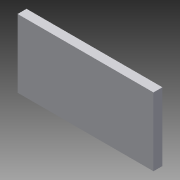
# Autodesk Inventor part: Lapangan2
Saved by Autodesk Inventor 2015 (Build 190159000, 159)
## iProperties
Created: 2015-01-29
Part Number: Lapangan2
Material: Generic
Document SubType Name: Modeling
Designer: Rafi Kurnia Putra
Density: 1 g/cm^3
Appearance: White
Author: Rafi Kurnia Putra
Autodesk Inventor part; units mm, degrees
ref_plane "YZ Plane" through (0, 0, 0) normal (1, 0, 0) x (0, 1, 0)
ref_plane "XZ Plane" through (0, 0, 0) normal (0, 1, 0) x (-1, 0, 0)
ref_plane "XY Plane" through (0, 0, 0) normal (0, 0, 1) x (1, 0, 0)
sketch "Sketch1" plane through (0, 0, 0) normal (0, 1, 0) x (-1, 0, 0)
  line L0 (2430, 1220) -> (0, 1220)
  line L1 (0, -1220) -> (2430, -1220)
  line L2 (2430, -1220) -> (2430, 1220)
  line L3 (2410, 1200) -> (2410, -1200)
  line L4 (10, 650) -> (10, 1200)
  line L5 (740, 150) -> (0, 150)
  line L6 (730, 170) -> (730, 740)
  line L7 (730, 740) -> (750, 740)
  line L8 (750, 740) -> (750, 150)
  line L9 (750, 150) -> (740, 150)
  line L10 (1210, 740) -> (1210, 270)
  line L11 (1230, 290) -> (1230, 740)
  line L12 (1230, 740) -> (1210, 740)
  line L13 (270, 630) -> (270, 650)
  line L14 (10, 1200) -> (2410, 1200)
  line L15 (0, -330) -> (10, -330)
  line L16 (0, -330) -> (10, -330) construction
  line L17 (10, -330) -> (10, -1200)
  line L18 (730, -1200) -> (730, -330)
  line L19 (750, -1200) -> (1600, -1200) construction
  line L20 (730, -330) -> (470, -330)
  line L21 (470, -330) -> (470, -310)
  line L22 (470, -310) -> (750, -310)
  line L23 (750, -310) -> (750, -1200)
  line L24 (2410, -1200) -> (750, -1200)
  line L25 (730, -1200) -> (10, -1200)
  line L26 (0, -1200) -> (730, -1200) construction
  line L27 (750, -1200) -> (870, -1200) construction
  line L28 (1210, 270) -> (1950, 270)
  line L29 (1210, 270) -> (1950, 270) construction
  line L30 (1950, 270) -> (1950, 290)
  line L31 (1950, 290) -> (1230, 290)
  line L32 (1950, -190) -> (1950, -740)
  line L33 (1950, -740) -> (1210, -740)
  line L34 (1210, -740) -> (1210, -190)
  line L35 (1210, -190) -> (1230, -190)
  line L36 (1210, -190) -> (1230, -190) construction
  line L37 (1230, -190) -> (1230, -720)
  line L38 (1230, -720) -> (1930, -720)
  line L39 (1930, -720) -> (1930, -210)
  line L40 (1930, -210) -> (1670, -210)
  line L41 (1670, -210) -> (1670, -190)
  line L42 (1670, -190) -> (1950, -190)
  line L43 (-2430, 1220) -> (0, 1220)
  line L44 (0, -1220) -> (-2430, -1220)
  line L45 (-2430, -1220) -> (-2430, 1220)
  line L46 (-2410, 1200) -> (-2410, -1200)
  line L47 (-10, 650) -> (-10, 1200)
  line L48 (-740, 150) -> (0, 150)
  line L49 (-730, 170) -> (-730, 740)
  line L50 (-730, 740) -> (-750, 740)
  line L51 (-750, 740) -> (-750, 150)
  line L52 (-750, 150) -> (-740, 150)
  line L53 (-1210, 740) -> (-1210, 270)
  line L54 (-1230, 290) -> (-1230, 740)
  line L55 (-1230, 740) -> (-1210, 740)
  line L56 (-270, 630) -> (-270, 650)
  line L57 (-10, 1200) -> (-2410, 1200)
  line L58 (0, -330) -> (-10, -330)
  line L59 (0, -330) -> (-10, -330) construction
  line L60 (-10, -330) -> (-10, -1200)
  line L61 (-730, -1200) -> (-730, -330)
  line L62 (-750, -1200) -> (-1600, -1200) construction
  line L63 (-730, -330) -> (-470, -330)
  line L64 (-470, -330) -> (-470, -310)
  line L65 (-470, -310) -> (-750, -310)
  line L66 (-750, -310) -> (-750, -1200)
  line L67 (-2410, -1200) -> (-750, -1200)
  line L68 (-730, -1200) -> (-10, -1200)
  line L69 (0, -1200) -> (-730, -1200) construction
  line L70 (-750, -1200) -> (-870, -1200) construction
  line L71 (-1210, 270) -> (-1950, 270)
  line L72 (-1210, 270) -> (-1950, 270) construction
  line L73 (-1950, 270) -> (-1950, 290)
  line L74 (-1950, 290) -> (-1230, 290)
  line L75 (-1950, -190) -> (-1950, -740)
  line L76 (-1950, -740) -> (-1210, -740)
  line L77 (-1210, -740) -> (-1210, -190)
  line L78 (-1210, -190) -> (-1230, -190)
  line L79 (-1210, -190) -> (-1230, -190) construction
  line L80 (-1230, -190) -> (-1230, -720)
  line L81 (-1230, -720) -> (-1930, -720)
  line L82 (-1930, -720) -> (-1930, -210)
  line L83 (-1930, -210) -> (-1670, -210)
  line L84 (-1670, -210) -> (-1670, -190)
  line L85 (-1670, -190) -> (-1950, -190)
  line L86 (270, 630) -> (-270, 630)
  line L87 (270, 650) -> (10, 650)
  line L88 (-10, 650) -> (-270, 650)
  line L89 (730, 170) -> (-730, 170)
  point P0 (0, 0)
  dimension "d274" = 4860
  dimension "d275" = 2440
  dimension "d276" = 2400
  dimension "d277" = 2400
  dimension "d278" = 720
  dimension "d279" = 450
  dimension "d280" = 20
  dimension "d281" = 470
  dimension "d282" = 740
  dimension "d283" = 20
  dimension "d284" = 700
  dimension "d285" = 510
  dimension "d286" = 260
  dimension "d287" = 20
  dimension "d288" = 280
  dimension "d289" = 550
  dimension "d290" = 740
  dimension "d291" = 550
  dimension "d292" = 20
  dimension "d293" = 530
  dimension "d294" = 890
  dimension "d295" = 280
  dimension "d296" = 20
  dimension "d297" = 260
  dimension "d298" = 870
  dimension "d300" = 870
  dimension "d301" = 20
  dimension "d302" = 550
  dimension "d303" = 260
  dimension "d304" = 20
  dimension "d305" = 540
  dimension "d306" = 570
  dimension "d307" = 20
  dimension "d308" = 590
  dimension "d309" = 1500
  dimension "d310" = 1460
  dimension "d311" = 2400
  dimension "d312" = 20
  dimension "d313" = 20
  dimension "d314" = 20
  dimension "d315" = 20
  dimension "d316" = 20
  dimension "d318" = 1660
  dimension "d319" = 20
  dimension "d320" = 720
  dimension "d324" = 20
  dimension "d330" = 720
  dimension "d331" = 740
  dimension "d332" = 470
  dimension "d333" = 20
  dimension "d334" = 20
  dimension "d336" = 530
  dimension "d337" = 510
  dimension "d338" = 260
  dimension "d339" = 20
  dimension "d341" = 550
  dimension "d343" = 550
  dimension "d346" = 870
  dimension "d352" = 460
  dimension "d353" = 460
  dimension "d356" = 460
  dimension "d358" = 460
  dimension "d359" = 460
  dimension "d364" = 460
  constraints: 180 end point, 36 parallel, 19 perpendicular, 12 horizontal, 4 collinear, 4 point on line, 2 vertical
  measures "d274" distance of L43.start L0.start
  measures "d275" distance of L1.end L0.start
  measures "d276" distance of L3.start L3.end
  measures "d277" distance of L4.end L3.start
  measures "d278" distance of L30.end L11.start
  measures "d279" distance of L11.start L11.end
  measures "d280" distance of L11.end L10.start
  measures "d281" distance of L10.start L10.end
  measures "d282" distance of L10.end L28.end
  measures "d283" distance of L28.end L30.end
  measures "d284" distance of L37.end L38.end
  measures "d285" distance of L38.end L39.end
  measures "d286" distance of L39.end L40.end
  measures "d287" distance of L40.end L41.end
  measures "d288" distance of L41.end L32.start
  measures "d289" distance of L32.start L32.end
  measures "d290" distance of L32.end L33.end
  measures "d291" distance of L33.end L34.end
  measures "d292" distance of L34.end L35.end
  measures "d293" distance of L35.end L37.end
  measures "d294" distance of L22.end L19.start
  measures "d295" distance of L21.end L22.end
  measures "d296" distance of L20.end L21.end
  measures "d297" distance of L18.end L20.end
  measures "d298" distance of L18.start L18.end
  measures "d300" distance of L15.end L17.end
  measures "d301" distance of L60.start L15.end
  measures "d302" distance of L4.start L4.end
  measures "d303" distance of L13.end L4.start
  measures "d304" distance of L13.start L13.end
  measures "d305" distance of L13.start L56.start
  measures "d306" distance of L6.start L6.end
  measures "d307" distance of L6.end L7.end
  measures "d308" distance of L7.end L8.end
  measures "d309" distance of L52.start L8.end
  measures "d310" distance of L6.start L49.start
  measures "d311" distance of L47.end L46.start
  measures "d312" distance between parallel lines of L47 L4
  measures "d313" distance between parallel lines of L3 L2
  measures "d314" distance between parallel lines of L45 L46
  measures "d315" distance between parallel lines of L0 L14
  measures "d316" distance between parallel lines of L24 L1
  measures "d318" distance of L3.end L19.start
  measures "d319" distance between parallel lines of L18 L23
  measures "d320" distance of L18.start L17.end
  measures "d324" distance of L50.start L50.end
  measures "d330" distance of L73.end L74.end
  measures "d331" distance of L71.start L73.start
  measures "d332" distance of L55.end L71.start
  measures "d333" distance of L55.start L55.end
  measures "d334" distance of L73.start L73.end
  measures "d336" distance of L80.start L81.start
  measures "d337" distance of L81.end L83.start
  measures "d338" distance of L83.start L84.start
  measures "d339" distance of L84.start L85.start
  measures "d341" distance of L85.end L76.start
  measures "d343" distance of L76.end L77.end
  measures "d346" distance of L60.start L60.end
  measures "d352" distance between parallel lines of L86 L89
  measures "d353" distance between parallel lines of L13 L6
  measures "d356" distance between parallel lines of L57 L50
  measures "d358" distance between parallel lines of L30 L3
  measures "d359" distance between parallel lines of L28 L42
  measures "d364" distance between parallel lines of L5 L22
extrude "Extrusion1" add sketch "Sketch1" along normal blind 20 contours L3 L24 L23 L22 L21 L20 L18 L25 L17 L15 L58 L60 L68 L61 L63 L64 L65 L66 L67 L46 L57 L47 L88 L56 L86 L13 L87 L4 L14
extrude "Extrusion2" add sketch "Sketch1" along normal blind 320
sketch "Sketch5" plane through (0, 20, 0) normal (0, 1, 0) x (1, 0, 0)
  line L0 (-10, 330) -> (10, 330)
  line L1 (-750, -150) -> (750, -150) projected
  line L2 (10, -130) -> (10, -150)
  line L3 (10, -150) -> (-10, -150)
  line L4 (-10, -150) -> (-10, -130)
  line L5 (-10, 330) -> (10, 330)
  line L6 (10, 330) -> (10, 310)
  line L7 (10, 310) -> (-10, 310)
  line L8 (-10, 310) -> (-10, 330)
  line L9 (-10, 310) -> (10, 310)
  line L10 (10, 310) -> (10, -150)
  line L11 (10, -150) -> (-10, -150)
  line L12 (-10, -150) -> (-10, 310)
  point P0 (0, 0)
  point P1 (-470, -150)
  point P2 (470, -150)
  dimension "d190" = 20
  dimension "d193" = 20
  dimension "d194" = 460
  constraints: 24 end point, 5 parallel, 3 horizontal, 2 perpendicular, 1 point on line
  measures "d190" distance of L5.end L6.end
  measures "d193" distance of L2.end L11.end
  measures "d194" distance of L9.end L2.end
extrude "Extrusion5" add sketch "Sketch5" along normal blind 300 contours L0 L6 L7 L8
body "Solid1"
